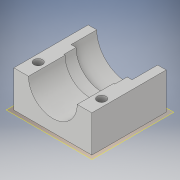
# Autodesk Inventor part: 5 Objektivhalterung oben 29112018
Saved by Autodesk Inventor 2018.3 (Build 223284000, 284)
## iProperties
Part Number: 5 Objektivhalterung oben 29112018
Material: Generisch
Document SubType Name: Modeling
Designer: pgmadmin
Density: 1 g/cm^3
Appearance: Vorgabe
Author: pgmadmin
Autodesk Inventor part; units mm, degrees
ref_plane "YZ Plane" through (0, 0, 0) normal (1, 0, 0) x (0, 1, 0)
ref_plane "XZ Plane" through (0, 0, 0) normal (0, 1, 0) x (-1, 0, 0)
sketch "Skizze1" plane through (0, 0, 0) normal (0, 0, 1) x (1, 0, 0)
  line L0 (-16, 20) -> (16, 20)
  line L1 (16, 20) -> (16, -20)
  line L2 (16, -20) -> (-16, -20)
  line L3 (-16, -20) -> (-16, 20)
  line L4 (-16, 20) -> (16, -20) construction
  line L5 (16, 20) -> (-16, -20) construction
  point P0 (0, 0)
  dimension "d0" = 32
  dimension "d1" = 40
  constraints: 12 end point, 2 midpoint, 2 parallel, 1 horizontal, 1 perpendicular
  measures "d0" distance of L1.end L2.end
  measures "d1" distance of L0.end L1.end
extrude "Extrusion1" add sketch "Skizze1" along normal blind 15
sketch "Skizze2" plane through (-16, -20, 0) normal (0, -1, 0) x (1, 0, 0)
  line L0 (0, 15) -> (32, 15) projected
  line L1 (0, 0) -> (0, 15) projected
  line L2 (32, 0) -> (0, 0) projected
  line L3 (32, 0) -> (32, 15) projected
  line L4 (32, 15) -> (0, 15) projected
  circle A0 centre (16, 15) radius 10
  point P0 (16, 0)
  dimension "d4" = 20
  constraints: 1 centre point, 1 midpoint
  measures "d4" diameter of A0
extrude "Extrusion2" cut sketch "Skizze2" against normal blind 15 contours A0 L0 | L0 A0
sketch "Skizze3" plane through (-16, -5, 0) normal (0, -1, 0) x (1, 0, 0)
  line L0 (0, 0) -> (0, 15) projected
  line L1 (32, 0) -> (0, 0) projected
  line L2 (32, 0) -> (32, 15) projected
  line L3 (26, 15) -> (32, 15) projected
  line L4 (0, 15) -> (6, 15) projected
  line L5 (6, 15) -> (26, 15) projected
  circle A0 centre (16, 15) radius 10.5
  point P0 (16, 0)
  dimension "d7" = 21
  constraints: 1 centre point, 1 midpoint
  measures "d7" diameter of A0
extrude "Extrusion3" cut sketch "Skizze3" against normal blind 5 contours A0 L3 L5 L4 | L4 L5 L3 A0
sketch "Skizze4" plane through (-16, 0, 0) normal (0, -1, 0) x (1, 0, 0)
  line L0 (5.5, 15) -> (26.5, 15) projected
  circle A0 centre (16, 15) radius 12.5
  point P0 (16, 0)
  dimension "d10" = 25
  constraints: 1 centre point, 1 midpoint
  measures "d10" diameter of A0
extrude "Extrusion4" cut sketch "Skizze4" against normal through all
sketch "Skizze5" plane through (0, 0, 15) normal (0, 0, 1) x (1, 0, 0)
  line L0 (-16, 20) -> (-16, -20) projected
  line L1 (-16, -20) -> (-10, -20) projected
  line L2 (-10, -20) -> (-10, -5) projected
  line L3 (10, -5) -> (10, -20) projected
  line L4 (10, -20) -> (16, -20) projected
  line L5 (16, -20) -> (16, 20) projected
  circle A0 centre (-13, -13) radius 1.8
  circle A1 centre (13, -13) radius 1.8
  point P0 (0, 0)
  dimension "d13" = 3.6
  dimension "d14" = 3.6
  dimension "d15" = 7
  dimension "d16" = 7
  dimension "d17" = 3
  dimension "d18" = 3
  constraints: 2 centre point
  measures "d13" diameter of A0
  measures "d14" diameter of A1
  measures "d15" distance from line of L1 A0.centre
  measures "d16" distance from line of L4 A1.centre
  measures "d17" distance from line of L5 A1.centre
  measures "d18" distance from line of L0 A0.centre
extrude "Extrusion5" cut sketch "Skizze5" against normal through all
sketch "Skizze6" plane through (0, 0, 0) normal (0, 0, 1) x (1, 0, 0)
  line L0 (16, 20) -> (16, -20) projected
  line L1 (-16, 20) -> (16, 20)
  line L2 (16, 20) -> (16, 10.5)
  line L3 (16, 10.5) -> (-16, 10.5)
  line L4 (-16, 10.5) -> (-16, 20)
  point P0 (0, 0)
  dimension "d21" = 9.5
  constraints: 8 end point, 2 parallel, 1 horizontal, 1 perpendicular, 1 point on line
  measures "d21" distance between parallel lines of L3 L1
extrude "Extrusion6" cut sketch "Skizze6" along normal blind 15
